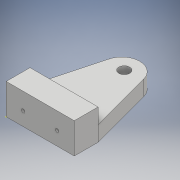
# Autodesk Inventor part: upper_deck_shaft_mount_for_AD
Saved by Autodesk Inventor 2019 (Build 230136000, 136)
## iProperties
Created: 2017-08-21
Part Number: upper_deck_shaft_mount_for_AD
Material: Generic
Document SubType Name: Modeling
Designer: ndz
Density: 1 g/cm^3
Appearance: Default
Author: ndz
Autodesk Inventor part; units mm, degrees
ref_plane "YZ Plane" through (0, 0, 0) normal (1, 0, 0) x (0, 1, 0)
ref_plane "XZ Plane" through (0, 0, 0) normal (0, 1, 0) x (-1, 0, 0)
ref_plane "XY Plane" through (0, 0, 0) normal (0, 0, 1) x (1, 0, 0)
sketch "Sketch1" plane through (0, 0, 0) normal (0, 0, 1) x (1, 0, 0)
  circle A0 centre (10, 24.7) radius 1.6
  line L0 (0, 0) -> (20.0001, 0)
  line L1 (0, 0) -> (0, 7)
  line L2 (20.0001, 0) -> (20.0001, 6.9998)
  line L3 (0, 7) -> (4.9176, 25.3526)
  line L4 (0, 7) -> (19, 7) construction
  line L5 (20.0001, 6.9998) -> (15.0825, 25.3524)
  line L6 (20.0001, 6.9998) -> (39.0001, 6.9998) construction
  arc A1 (15.0825, 25.3524) -> (4.9176, 25.3526) centre (10, 23.9906) ccw
  dimension "d17" = 7
  dimension "d18" = 6.9998
  dimension "d19" = 24.7
  dimension "d23" = 90
  dimension "d24" = 90
  dimension "d25" = 10
  dimension "d26" = 19
  dimension "d27" = 75
  dimension "d28" = 19
  dimension "d29" = 105
  dimension "d30" = 10
  constraints: 14 end point, 2 centre point, 2 equal length, 2 horizontal, 2 point on circle, 1 tangent, 1 vertical
  measures "d17" distance of L0.start L1.end
  measures "d18" distance of L0.end L2.end
  measures "d19" distance from line of A0.centre L0
  measures "d23" angle of L0 L1
  measures "d24" angle of L0 L2
  measures "d25" distance from line of L1 A0.centre
  measures "d26" distance of L1.end L3.end
  measures "d27" angle of L4 L3
  measures "d28" distance of L2.end L5.end
  measures "d29" angle of L6 L5
  measures "d30" distance from line of L1 A1.centre
sketch "Sketch3" plane through (0, 0, 0) normal (0, 0, 1) x (1, 0, 0)
  point P0 (0, 0)
extrude "Extrusion1" add sketch "Sketch1" along normal blind 4.5
sketch "Sketch4" plane through (0, 0, 4.5) normal (0, 0, 1) x (1, 0, 0)
  line L0 (0, 7) -> (0, 0) projected
  line L1 (20.0001, 0) -> (20.0001, 6.9998) projected
  line L2 (0, 0) -> (20.0001, 0)
  line L3 (20.0001, 0) -> (20.0001, 6.9998)
  line L4 (3.884, 22.9404) -> (-0.0481, 7.0119) projected
  line L5 (20.0001, 6.9998) -> (0, 6.9998)
  line L6 (0, 7) -> (0, 0)
  constraints: 8 end point, 3 perpendicular, 1 collinear
extrude "Extrusion2" add sketch "Sketch4" along normal blind 4.5
sketch "Sketch5" plane through (0, 0, 0) normal (0, -1, 0) x (1, 0, 0)
  circle A0 centre (5, 4) radius 0.5
  circle A1 centre (15, 4) radius 0.5
  line L0 (0, 0) -> (20.0001, 0) projected
  line L1 (0, 9) -> (20.0001, 9) projected
  dimension "d13" = 1
  dimension "d14" = 1
  dimension "d33" = 5
  dimension "d34" = 5
  constraints: 2 centre point
  measures "d13" diameter of A0
  measures "d14" diameter of A1
  measures "d33" distance from line of L1 A0.centre
  measures "d34" distance from line of L1 A1.centre
extrude "Extrusion3" cut sketch "Sketch5" against normal blind 5.5
body "Solid1"
